Autodesk Inventor part; units mm, degrees
(part 4 of 4)
  line L2182 (8.826805, 207.614987) -> (8.805299, 207.663374)
  line L2183 (8.805299, 207.663374) -> (8.779762, 207.713777)
  line L2184 (8.779762, 207.713777) -> (8.754896, 207.764852)
  line L2185 (8.754896, 207.764852) -> (8.711214, 207.829368)
  line L2186 (8.711214, 207.829368) -> (8.667531, 207.894556)
  line L2187 (8.667531, 207.894556) -> (8.617128, 207.95168)
  line L2188 (8.617128, 207.95168) -> (8.566053, 208.008803)
  line L2189 (8.566053, 208.008803) -> (8.514306, 208.053158)
  line L2190 (8.514306, 208.053158) -> (8.462558, 208.096841)
  line L2191 (8.462558, 208.096841) -> (8.39401, 208.141867)
  line L2192 (8.39401, 208.141867) -> (8.32479, 208.187566)
  line L2193 (8.32479, 208.187566) -> (8.246161, 208.224528)
  line L2194 (8.246161, 208.224528) -> (8.166861, 208.261491)
  line L2195 (8.166861, 208.261491) -> (8.105033, 208.281652)
  line L2196 (8.105033, 208.281652) -> (8.042533, 208.302485)
  line L2197 (8.042533, 208.302485) -> (7.965249, 208.319286)
  line L2198 (7.965249, 208.319286) -> (7.887964, 208.336087)
  line L2199 (7.887964, 208.336087) -> (7.82748, 208.344152)
  line L2200 (7.82748, 208.344152) -> (7.766997, 208.352216)
  line L2201 (7.766997, 208.352216) -> (7.434335, 208.351544)
  line L2202 (7.434335, 208.351544) -> (7.101674, 208.3502)
  line L2203 (7.101674, 208.3502) -> (7.039174, 208.339447)
  line L2204 (7.039174, 208.339447) -> (6.977347, 208.328695)
  line L2205 (6.977347, 208.328695) -> (6.902078, 208.309206)
  line L2206 (6.902078, 208.309206) -> (6.826137, 208.289716)
  line L2207 (6.826137, 208.289716) -> (6.769014, 208.269555)
  line L2208 (6.769014, 208.269555) -> (6.71189, 208.249394)
  line L2209 (6.71189, 208.249394) -> (6.627885, 208.205711)
  line L2210 (6.627885, 208.205711) -> (6.54388, 208.162701)
  line L2211 (6.54388, 208.162701) -> (6.500197, 208.132459)
  line L2212 (6.500197, 208.132459) -> (6.456515, 208.102217)
  line L2213 (6.456515, 208.102217) -> (6.406784, 208.059207)
  line L2214 (6.406784, 208.059207) -> (6.357053, 208.016196)
  line L2215 (6.357053, 208.016196) -> (6.305978, 207.961761)
  line L2216 (6.305978, 207.961761) -> (6.254903, 207.906653)
  line L2217 (6.254903, 207.906653) -> (6.2045, 207.830713)
  line L2218 (6.2045, 207.830713) -> (6.154097, 207.7541)
  line L2219 (6.154097, 207.7541) -> (6.123183, 207.690256)
  line L2220 (6.123183, 207.690256) -> (6.092269, 207.626412)
  line L2221 (6.092269, 207.626412) -> (6.070764, 207.569289)
  line L2222 (6.070764, 207.569289) -> (6.04993, 207.512165)
  line L2223 (6.04993, 207.512165) -> (6.032457, 207.450337)
  line L2224 (6.032457, 207.450337) -> (6.014984, 207.38851)
  line L2225 (6.014984, 207.38851) -> (6.000871, 207.302489)
  line L2226 (6.000871, 207.302489) -> (5.986086, 207.216467)
  line L2227 (5.986086, 207.216467) -> (5.98071, 207.129102)
  line L2228 (5.98071, 207.129102) -> (5.974662, 207.041737)
  line L2229 (5.974662, 207.041737) -> (5.975334, 206.172788)
  line L2230 (5.975334, 206.172788) -> (5.975332, 206.172784)
  line L2231 (6.750194, 206.609611) -> (6.752883, 207.108937)
  line L2232 (6.752883, 207.108937) -> (6.764307, 207.149259)
  line L2233 (6.764307, 207.149259) -> (6.775732, 207.189582)
  line L2234 (6.775732, 207.189582) -> (6.802614, 207.244017)
  line L2235 (6.802614, 207.244017) -> (6.828823, 207.298452)
  line L2236 (6.828823, 207.298452) -> (6.867801, 207.341463)
  line L2237 (6.867801, 207.341463) -> (6.906108, 207.384473)
  line L2238 (6.906108, 207.384473) -> (6.932989, 207.405307)
  line L2239 (6.932989, 207.405307) -> (6.960543, 207.425468)
  line L2240 (6.960543, 207.425468) -> (6.997505, 207.446973)
  line L2241 (6.997505, 207.446973) -> (7.034468, 207.467806)
  line L2242 (7.034468, 207.467806) -> (7.096967, 207.487968)
  line L2243 (7.096967, 207.487968) -> (7.158795, 207.508801)
  line L2244 (7.158795, 207.508801) -> (7.211214, 207.516193)
  line L2245 (7.211214, 207.516193) -> (7.262961, 207.523586)
  line L2246 (7.262961, 207.523586) -> (7.501536, 207.520898)
  line L2247 (7.501536, 207.520898) -> (7.740111, 207.518209)
  line L2248 (7.740111, 207.518209) -> (7.793874, 207.502752)
  line L2249 (7.793874, 207.502752) -> (7.847637, 207.487968)
  line L2250 (7.847637, 207.487968) -> (7.910809, 207.457054)
  line L2251 (7.910809, 207.457054) -> (7.973308, 207.42614)
  line L2252 (7.973308, 207.42614) -> (8.025056, 207.375065)
  line L2253 (8.025056, 207.375065) -> (8.076131, 207.32399)
  line L2254 (8.076131, 207.32399) -> (8.101668, 207.280307)
  line L2255 (8.101668, 207.280307) -> (8.127206, 207.236624)
  line L2256 (8.127206, 207.236624) -> (8.142663, 207.186221)
  line L2257 (8.142663, 207.186221) -> (8.158792, 207.135818)
  line L2258 (8.158792, 207.135818) -> (8.166184, 207.077351)
  line L2259 (8.166184, 207.077351) -> (8.173577, 207.018211)
  line L2260 (8.173577, 207.018211) -> (8.173577, 206.564583)
  line L2261 (8.173577, 206.564583) -> (8.173577, 206.110954)
  line L2262 (8.173577, 206.110954) -> (7.461214, 206.110954)
  line L2263 (7.461214, 206.110954) -> (6.748177, 206.110954)
  line L2264 (6.748177, 206.110954) -> (6.750193, 206.609609)
  line L2265 (6.750193, 206.609609) -> (6.750194, 206.609611)
  point P0 (0, 0)
  constraints: 4532 end point
equation "\"d50\" = 2 * d49"
